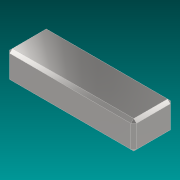
# Autodesk Inventor part: spie
Saved by Autodesk Inventor 2020.2 (Build 242310000, 310)
## iProperties
Created: 2020-05-14
Part Number: spie
Material: Stainless Steel
Document SubType Name: Modeling
Designer: Svend
Density: 8 g/cm^3
Appearance: Semi-Polished
Author: Svend
Autodesk Inventor part; units mm, degrees
ref_plane "YZ Plane" through (0, 0, 0) normal (1, 0, 0) x (0, 1, 0)
ref_plane "XZ Plane" through (0, 0, 0) normal (0, 1, 0) x (-1, 0, 0)
ref_plane "XY Plane" through (0, 0, 0) normal (0, 0, 1) x (1, 0, 0)
sketch "Sketch1" plane through (0, 0, 0) normal (0, 0, 1) x (1, 0, 0)
  line L0 (0, 0) -> (9, 0)
  line L1 (9, 0) -> (9, 2)
  line L2 (9, 2) -> (0, 2)
  line L3 (0, 2) -> (0, 0)
  dimension "d0" = 9
  dimension "d1" = 2
  constraints: 8 end point, 2 parallel, 1 horizontal, 1 perpendicular
  measures "d0" distance of L2.end L1.end
  measures "d1" distance of L1.end L0.end
extrude "Extrusion1" add sketch "Sketch1" along normal blind 2.8
chamfer "Chamfer1" distance 0.2 angle 45 12 edges at (4.5, 0, 2.8) (4.5, 0, 0) (9, 0, 1.4) (9, 1, 2.8) (9, 1, 0) (9, 2, 1.4) (4.5, 2, 2.8) (4.5, 2, 0) (0, 2, 1.4) (0, 1, 2.8) (0, 0, 1.4) (0, 1, 0)
body "Solid1"
